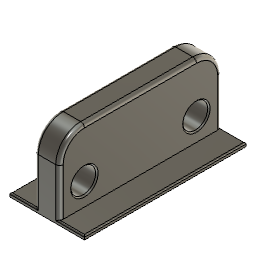
Filament storage (Autodesk Fusion 360 design; units mm, degrees)
Autodesk Fusion 360 part; units mm, degrees
sketch "Sketch1" plane through (0, 0, 0) normal (1, 0, 0) x (0, 1, 0)
  line L0 (-80, 0) -> (50, 0)
  line L1 (50, 0) -> (50, 60)
  line L2 (50, 60) -> (-80, 60)
  line L3 (-80, 60) -> (-80, 0)
  dimension "d1" = 130
  dimension "d2" = 60
  constraint horizontal L0
  constraint vertical L1
  constraint horizontal L2
  constraint vertical L3
  measures "d1" distance of L0.start L0.end
  measures "d2" distance of L0.start L2.end
extrude "Extrude1" add sketch "Sketch1" along normal blind 20
fillet "Fillet1" radius 20 2 edges at (10, -80, 60) (10, 50, 60)
sketch "Sketch2" plane through (20, 0, 0) normal (1, 0, 0) x (0, 1, 0)
  circle A0 centre (-60, 20) radius 10
  circle A1 centre (30, 20) radius 10
  arc A2 (50, 40) -> (30, 60) centre (30, 40) ccw
  line L0 (30, 60) -> (-60, 60)
  arc A3 (-60, 60) -> (-80, 40) centre (-60, 40) ccw
  line L1 (-80, 40) -> (-80, 0)
  line L2 (-80, 0) -> (50, 0)
  line L3 (50, 0) -> (50, 40)
  dimension "d11" = 20
  dimension "d14" = 90
  dimension "d15" = 0
  measures "d11" diameter of A0
extrude "Extrude2" cut sketch "Sketch2" against normal blind 20 contours A0 | A1
chamfer "Chamfer1" distance 1 angle 45 4 edges at (20, -69.3233, 23.6162) (20, 20.6767, 23.6162) (0, 20.6767, 16.3838) (0, -69.3233, 16.3838)
sketch "Sketch3" plane through (0, 0, 0) normal (-1, 0, 0) x (0, -1, 0)
  circle A0 centre (-30, 20) radius 11
  arc A1 (-30, 60) -> (-50, 40) centre (-30, 40) ccw
  line L0 (-50, 40) -> (-50, 0)
  line L1 (-50, 0) -> (80, 0)
  line L2 (80, 0) -> (80, 40)
  arc A2 (80, 40) -> (60, 60) centre (60, 40) ccw
  line L3 (60, 60) -> (-30, 60)
  circle A3 centre (60, 20) radius 11
  line L4 (-50, 0) -> (80, 0)
  line L5 (80, 0) -> (80, 2)
  line L6 (80, 2) -> (-50, 2)
  line L7 (-50, 2) -> (-50, 0)
  dimension "d19" = 2
  constraint horizontal L4
  constraint vertical L5
  constraint horizontal L6
  constraint vertical L7
  constraint coincident L0.end L1.start
  measures "d19" distance of L0.end L6.end
extrude "Extrude3" add sketch "Sketch3" along normal blind 20 contours L0 L1 L2 L4 L5 L6 L7
extrude "Extrude4" add 1 faces at (-20, 6.6667, 0.6667) along direction (1, 0, 0) blind 60
fillet "Fillet4" radius 3 10 edges at (20, 50, 21) (20, 44.1421, 54.1421) (20, -15, 60) (20, -74.1421, 54.1421) (20, -80, 21) (0, 50, 21) (0, 44.1421, 54.1421) (0, -15, 60) (0, -74.1421, 54.1421) (0, -80, 21)
fillet "Fillet5" radius 1 6 edges at (40, -15, 2) (28.5, 50, 2) (28.5, -80, 2) (-8.5, 50, 2) (-20, -15, 2) (-8.5, -80, 2)
extrude "Extrude5" add 1 faces at (0, 6.6667, 0) along direction (0, 0, -1) blind 1
